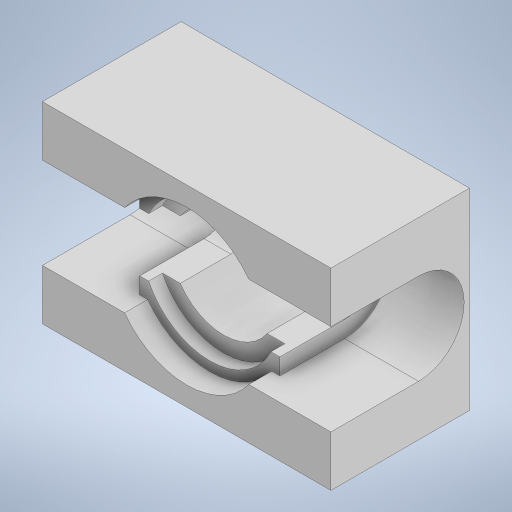
# Autodesk Inventor part: Ball Valve Mount
Saved by Autodesk Inventor 2024 (Build 280153000, 153)
## iProperties
Created: 2024-11-25
Part Number: Ball Valve Mount
Material: Generic
Document SubType Name: Modeling
Designer: Tommy Rohmann
Density: 1 g/cm^3
Appearance: Default
Author: Tommy Rohmann
Autodesk Inventor part; units mm, degrees
ref_plane "YZ Plane" through (0, 0, 0) normal (1, 0, 0) x (0, 1, 0)
ref_plane "XZ Plane" through (0, 0, 0) normal (0, 1, 0) x (-1, 0, 0)
ref_plane "XY Plane" through (0, 0, 0) normal (0, 0, 1) x (1, 0, 0)
sketch "Sketch1" plane through (0, 0, 0) normal (0, 0, 1) x (1, 0, 0)
  circle A0 centre (0, 0) radius 8.636
  circle A1 centre (0, 0) radius 11.176
  line L0 (11.5697, -15.875) -> (-11.5697, -15.875)
  line L1 (-11.5697, -15.875) -> (-11.5697, 15.875)
  line L2 (-11.5697, 15.875) -> (11.5697, 15.875)
  line L3 (11.5697, 15.875) -> (11.5697, -15.875)
  line L4 (11.5697, -15.875) -> (-11.5697, 15.875) construction
  line L5 (-11.5697, -15.875) -> (11.5697, 15.875) construction
  line L6 (0, 15.875) -> (0, -15.875)
  dimension "d0" = 17.272
  dimension "d1" = 22.352
  dimension "d2" = 23.1394
  dimension "d3" = 31.75
  constraints: 14 end point, 4 midpoint, 2 centre point, 2 coincident, 2 parallel, 1 horizontal, 1 perpendicular
  measures "d0" diameter of A0
  measures "d1" diameter of A1
  measures "d2" distance of L0.start L0.end
  measures "d3" distance of L0.end L1.end
extrude "Extrusion1" add sketch "Sketch1" against normal blind 19.05 contours L6 A0 | A0 L6 A1 | A1 L6 L0 L1 L2 picked at (-2.3691, -1.6353) picked at (-10.254, 0.347)
extrude "Extrusion2" cut sketch "Sketch1" against normal blind 28.321 contours A0 L6 | L6 A0
extrude "Extrusion3" cut sketch "Sketch1" against normal blind 2.286 contours A0 L6 A1 | A0 L6 A1
sketch "Sketch3" plane through (-11.5697, -15.875, 0) normal (-1, 0, 0) x (0, 0, 1)
  line L0 (0, 0) -> (-19.05, 0) projected
  line L1 (0, 31.75) -> (0, 0) projected
  line L2 (0, 31.75) -> (-19.05, 31.75) projected
  line L3 (-19.05, 0) -> (-19.05, 31.75) projected
  line L4 (0, 0) -> (-19.05, 0) projected
  line L5 (-19.05, 15.875) -> (0, 15.875)
  circle A0 centre (-10.6426, 15.875) radius 4.826
  circle A1 centre (-10.6426, 15.875) radius 7.5184
  line L6 (-10.6426, 11.049) -> (0, 11.049)
  line L7 (-10.6426, 8.3566) -> (0, 8.3566)
  line L8 (0, 0) -> (0, 31.75) projected
  line L9 (-10.6426, 20.701) -> (0, 20.701)
  line L10 (-10.6426, 23.3934) -> (0, 23.3934)
  point P0 (0, 8.3566)
  dimension "d10" = 9.652
  dimension "d11" = 15.0368
  dimension "d12" = 10.6426
  constraints: 10 end point, 5 point on line, 4 point on circle, 4 tangent, 3 perpendicular, 2 centre point, 1 coincident, 1 horizontal, 1 midpoint, 1 parallel
  measures "d10" diameter of A0
  measures "d11" diameter of A1
  measures "d12" distance from line of L1 A0.centre
extrude "Extrusion4" add sketch "Sketch3" along normal blind 12.2174 contours L0 L3 L5 A1 L7 L1 | L3 L2 L1 L10 A1 L5
extrude "Extrusion5" cut sketch "Sketch3" against normal blind 34.4424 contours L6 A1 L5 L1 | L5 A1 L9 L1 | L6 A0 L5 A1 | A0 L5 | L5 A0 | L5 A0 L9 A1 picked at (-4.1293, 14.94) picked at (-4.1293, 16.81)
sketch "Sketch4" plane through (0, 0, 0) normal (0, 0, 1) x (1, 0, 0)
  line L0 (-11.5697, 4.826) -> (-10.0803, 4.826) projected
  arc A0 (0, 11.176) -> (-10.0803, 4.826) centre (0, 0) ccw projected
  line L1 (0, 11.176) -> (0, 15.875) projected
  line L2 (0, 15.875) -> (-23.7871, 15.875) projected
  line L3 (-23.7871, 7.5184) -> (-23.7871, 15.875) projected
  line L4 (-11.5697, 7.5184) -> (-23.7871, 7.5184) projected
  line L5 (-11.5697, 7.5184) -> (-11.5697, 4.826) projected
  line L6 (-10.0803, -4.826) -> (-11.5697, -4.826) projected
  line L7 (-11.5697, -4.826) -> (-11.5697, -7.5184) projected
  line L8 (-11.5697, -7.5184) -> (-23.7871, -7.5184) projected
  line L9 (-23.7871, -15.875) -> (-23.7871, -7.5184) projected
  line L10 (-23.7871, -15.875) -> (0, -15.875) projected
  line L11 (0, -15.875) -> (0, -11.176) projected
  arc A1 (-10.0803, -4.826) -> (0, -11.176) centre (0, 0) ccw projected
  circle A2 centre (0, 0) radius 12.7
  line L12 (-23.7871, 7.5184) -> (7.145, 7.5184)
  line L13 (-23.7871, -7.5184) -> (8.7608, -7.5184)
  point P0 (0, -12.7)
  point P1 (-11.5697, -5.2376)
  point P2 (-11.5697, 5.2376)
  point P3 (0, 12.7)
  point P4 (-10.2354, 7.5184)
  point P5 (-10.2354, -7.5184)
  dimension "d17" = 25.4
  constraints: 4 end point, 2 horizontal, 1 centre point, 1 coincident
  measures "d17" diameter of A2
extrude "Extrusion6" add sketch "Sketch4" along normal blind 3.81 contours L4 L3 L2 L1 A2 L12 | L13 A2 L11 L10 L9 L8
mirror "Mirror1" about plane through (0, 0, 0) normal (1, 0, 0)
body "Solid1"
